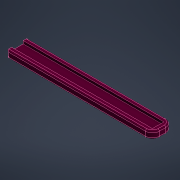
# Autodesk Inventor part: ArmRestCushion
Saved by Autodesk Inventor 2021 (Build 250183000, 183)
## iProperties
Created: 2021-01-30
Part Number: ArmRestCushion
Material: Generic
Document SubType Name: Modeling
Designer: argon
Density: 1 g/cm^3
Appearance: Sky Blue Medium
Author: argon
Autodesk Inventor part; units mm, degrees
ref_plane "YZ Plane" through (0, 0, 0) normal (1, 0, 0) x (0, 1, 0)
ref_plane "XZ Plane" through (0, 0, 0) normal (0, 1, 0) x (-1, 0, 0)
ref_plane "XY Plane" through (0, 0, 0) normal (0, 0, 1) x (1, 0, 0)
sketch "Sketch1" plane through (0, 0, 0) normal (0, 1, 0) x (-1, 0, 0)
  line L0 (243.2455, 20) -> (-243.2455, 20)
  line L1 (-243.2455, 20) -> (-243.2455, -20)
  line L2 (-243.2455, -20) -> (243.2455, -20)
  line L3 (243.2455, -20) -> (243.2455, 20)
  line L4 (243.2455, 20) -> (-243.2455, -20) construction
  line L5 (-243.2455, 20) -> (243.2455, -20) construction
  line L6 (243.2455, 35) -> (-258.2455, 35)
  line L7 (-258.2455, 35) -> (-258.2455, -35)
  line L8 (-258.2455, -35) -> (243.2455, -35)
  line L9 (243.2455, -35) -> (243.2455, 35)
  line L10 (243.2455, 35) -> (-258.2455, -35) construction
  line L11 (-258.2455, 35) -> (243.2455, -35) construction
  point P0 (0, 0)
  point P1 (-7.5, 0)
  point P2 (243.2455, 20)
  point P3 (243.2455, -20)
  dimension "d0" = 486.491
  dimension "d1" = 40
  dimension "d2" = 15
  dimension "d3" = 15
  constraints: 24 end point, 4 midpoint, 4 parallel, 2 horizontal, 2 perpendicular, 1 collinear, 1 horizontal alignment
  measures "d0" distance of L0.start L0.end
  measures "d1" distance of L2.end L0.start
  measures "d2" distance between parallel lines of L7 L1
  measures "d3" distance between parallel lines of L2 L8
extrude "Extrusion1" add sketch "Sketch1" along normal blind 15 contours L3 L2 L1 L0
extrude "Extrusion2" add sketch "Sketch1" along normal blind 25 contours L0 L1 L2 L9 L8 L7 L6
fillet "Fillet1" radius 24 2 edges at (258.2455, 12.5, -35) (258.2455, 12.5, 35)
fillet "Fillet2" radius 5 11 edges at (258.2455, 0, 0) (-4.5, 0, 35) (-4.5, 0, -35) (-243.2455, 12.5, -35) (-243.2455, 12.5, 35) (251.2161, 25, -27.9706) (258.2455, 25, 0) (251.2161, 25, 27.9706) (-4.5, 25, 35) (-4.5, 25, -35) (-243.2455, 0, 0)
body "Solid1"
